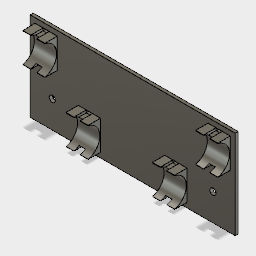
Solenoid Housing (Autodesk Fusion 360 design; units mm, degrees)
Autodesk Fusion 360 part; units mm, degrees
box "BoxPrimitive1" add length 60 width 90 height 10 placed x (0, 1, 0) y (-1, 0, 0) z (0, 0, 1) at (100, 10, 0) makes body 1 in component "SolenoidHousing"
box "BoxPrimitive1'" add length 24 width 16 height 10 placed x (0, -1, 0) y (1, 0, 0) z (0, 0, 1) at (20, 60, 10) separate body makes body 2 in component "mounting"
hole "Hole1" at (36, 47.925, 22.5451) direction (-1, 0, 0) diameter 24 depth 20 tip angle 118 bodies 2 in component "mounting"
sketch "Sketch2" plane through (0, 36, 0) normal (0, -1, 0) x (1, 0, 0) in component "mounting"
  line L0 (20, 20) -> (20, 10)
  line L1 (20, 10) -> (36, 10)
  line L2 (36, 10) -> (36, 20)
  line L3 (36, 20) -> (20, 20)
  line L4 (28, 10) -> (28, 20) construction
  line L5 (28, 20) -> (25.5, 20)
  dimension "d14" = 2.5
  constraint midpoint L1
  constraint midpoint L3
box "BoxPrimitive2" cut length 10 width 5 height -2 placed x (0, 0, 1) y (-1, 0, 0) z (0, -1, 0) at (29.5, 36, 10) bodies 2 in component "mounting"
box "BoxPrimitive3" cut length 10 width 5 height -2 placed x (0, 0, -1) y (-1, 0, 0) z (0, 1, 0) at (29.5, 60, 20) bodies 2 in component "mounting"
move_face "OffsetFaces1" offset 2 1 faces at (20, 57.177, 12.3342) on bodies 2 in component "mounting"
box "BoxPrimitive1''" add length 24 width 16 height 10 placed x (0, -1, 0) y (1, 0, 0) z (0, 0, 1) at (20, 60, 10) separate body makes body 3 in component "mounting (1)"
hole "Hole1'" at (36, 47.925, 22.5451) direction (-1, 0, 0) diameter 24 depth 20 tip angle 118 bodies 3 in component "mounting (1)"
sketch "Sketch2 (2)" plane through (0, 36, 0) normal (0, -1, 0) x (1, 0, 0) in component "mounting (1)"
  line L0 (20, 20) -> (20, 10)
  line L1 (20, 10) -> (36, 10)
  line L2 (36, 10) -> (36, 20)
  line L3 (36, 20) -> (20, 20)
  line L4 (28, 10) -> (28, 20) construction
  line L5 (28, 20) -> (25.5, 20)
  dimension "d14_1" = 2.5
  constraint midpoint L1
  constraint midpoint L3
box "BoxPrimitive2'" cut length 10 width 5 height -2 placed x (0, 0, 1) y (-1, 0, 0) z (0, -1, 0) at (29.5, 36, 10) bodies 3 in component "mounting (1)"
box "BoxPrimitive3'" cut length 10 width 5 height -2 placed x (0, 0, -1) y (-1, 0, 0) z (0, 1, 0) at (29.5, 60, 20) bodies 3 in component "mounting (1)"
move_face "OffsetFaces1'" offset 2 1 faces at (20, 57.177, 12.3342) on bodies 3 in component "mounting (1)"
box "BoxPrimitive1'''" add length 24 width 16 height 10 placed x (0, -1, 0) y (1, 0, 0) z (0, 0, 1) at (20, 60, 10) separate body makes body 4 in component "mounting (2)"
hole "Hole1''" at (36, 47.925, 22.5451) direction (-1, 0, 0) diameter 24 depth 20 tip angle 118 bodies 4 in component "mounting (2)"
sketch "Sketch2 (3)" plane through (0, 36, 0) normal (0, -1, 0) x (1, 0, 0) in component "mounting (2)"
  line L0 (20, 20) -> (20, 10)
  line L1 (20, 10) -> (36, 10)
  line L2 (36, 10) -> (36, 20)
  line L3 (36, 20) -> (20, 20)
  line L4 (28, 10) -> (28, 20) construction
  line L5 (28, 20) -> (25.5, 20)
  dimension "d14_1" = 2.5
  constraint midpoint L1
  constraint midpoint L3
box "BoxPrimitive2''" cut length 10 width 5 height -2 placed x (0, 0, 1) y (-1, 0, 0) z (0, -1, 0) at (29.5, 36, 10) bodies 4 in component "mounting (2)"
box "BoxPrimitive3''" cut length 10 width 5 height -2 placed x (0, 0, -1) y (-1, 0, 0) z (0, 1, 0) at (29.5, 60, 20) bodies 4 in component "mounting (2)"
move_face "OffsetFaces1''" offset 2 1 faces at (20, 57.177, 12.3342) on bodies 4 in component "mounting (2)"
move_face "OffsetFaces1'''" offset 25 1 faces at (100, 50, 3.3333) on bodies 1 in component "SolenoidHousing"
move_face "OffsetFaces2" offset 50 1 faces at (10, 50, 3.3333) on bodies 1 in component "SolenoidHousing"
move_face "OffsetFaces3" offset -2 1 faces at (70, 10, 3.3333) on bodies 1 in component "SolenoidHousing"
move_face "OffsetFaces4" offset 13 1 faces at (70, 70, 3.3333) on bodies 1 in component "SolenoidHousing"
move_face "OffsetFaces5" offset 1 1 faces at (-40, 59.3333, 3.3333) on bodies 1 in component "SolenoidHousing"
move_face "OffsetFaces6" offset 1 1 faces at (69.6667, 83, 3.3333) on bodies 1 in component "SolenoidHousing"
move_face "OffsetFaces7" offset -7.5 1 faces at (14.3333, 36, 0) on bodies 1 in component "SolenoidHousing"
sketch "Sketch2 (4)" plane through (0, 0, 10) normal (0, 0, 1) x (1, 0, 0) in component "SolenoidHousing"
  line L0 (125, 84) -> (-41, 84)
  line L1 (-41, 84) -> (-41, 12)
  line L2 (-41, 12) -> (125, 12)
  line L3 (125, 12) -> (125, 84)
  line L4 (125, 12) -> (125, 34)
  line L5 (125, 34) -> (-41, 34) construction
  line L6 (42, 34) -> (107, 34)
  line L7 (42, 34) -> (-23, 34)
  dimension "d33" = 22
  dimension "d34" = 65
  dimension "d35" = 65
  constraint coincident L1
  constraint perpendicular L1 L5
  constraint midpoint L5
  constraint coincident L5
  constraint parallel L5 L6
sketch "Sketch3" plane through (0, 0, 10) normal (0, 0, 1) x (1, 0, 0) in component "SolenoidHousing"
hole "Hole1'''" at (-23, 34, 10) direction (0, 0, -1) diameter 5 depth 5 tip angle 118 bodies 1 in component "SolenoidHousing"
hole "Hole2" at (107, 34, 10) direction (0, 0, -1) diameter 5 depth 5 tip angle 118 bodies 1 in component "SolenoidHousing"
box "BoxPrimitive2'''" cut length 2 width 5 height -2 placed x (0, -1, 0) y (1, 0, 0) z (0, 0, 1) at (-30.5, 80, 10) bodies 1 in component "SolenoidHousing"
box "BoxPrimitive3'''" cut length 2 width 5 height -5 placed x (0, -1, 0) y (1, 0, 0) z (0, 0, 1) at (-30.5, 80, 10) bodies 1 in component "SolenoidHousing"
box "BoxPrimitive4" cut length 2 width 5 height -5 placed x (0, -1, 0) y (1, 0, 0) z (0, 0, 1) at (-30.5, 58, 10) bodies 1 in component "SolenoidHousing"
box "BoxPrimitive5" cut length 2 width 5 height -5 placed x (0, -1, 0) y (1, 0, 0) z (0, 0, 1) at (4.5, 40, 10) bodies 1 in component "SolenoidHousing"
box "BoxPrimitive6" cut length 2 width 5 height -5 placed x (0, -1, 0) y (1, 0, 0) z (0, 0, 1) at (4.5, 18, 10) bodies 1 in component "SolenoidHousing"
box "BoxPrimitive7" cut length 2 width 5 height -5 placed x (0, -1, 0) y (1, 0, 0) z (0, 0, 1) at (74.5, 18, 10) bodies 1 in component "SolenoidHousing"
box "BoxPrimitive8" cut length 2 width 5 height -5 placed x (0, -1, 0) y (1, 0, 0) z (0, 0, 1) at (74.5, 40, 10) bodies 1 in component "SolenoidHousing"
box "BoxPrimitive9" cut length 2 width 5 height -5 placed x (0, -1, 0) y (1, 0, 0) z (0, 0, 1) at (109.5, 80, 10) bodies 1 in component "SolenoidHousing"
box "BoxPrimitive10" cut length 2 width 5 height -5 placed x (0, 1, 0) y (-1, 0, 0) z (0, 0, 1) at (114.5, 56, 10) bodies 1 in component "SolenoidHousing"
component "SolenoidHousing" placed x (1, 0, 0) y (0, 1, 0) z (0, 0, 1) at (0, 0, 0)
component "mounting" placed x (1, 0, 0) y (0, 1, 0) z (0, 0, 1) at (50, -20, 0) in component "SolenoidHousing"
component "mounting (1)" placed x (1, 0, 0) y (0, 1, 0) z (0, 0, 1) at (85, 20, 0) in component "SolenoidHousing"
component "mounting (2)" placed x (1, 0, 0) y (0, 1, 0) z (0, 0, 1) at (-20, -20, 0) in component "SolenoidHousing"
component "mounting" placed x (1, 0, 0) y (0, 1, 0) z (0, 0, 1) at (-55, 20, 0) in component "SolenoidHousing"
